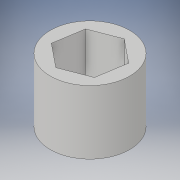
# Autodesk Inventor part: wheel spacer
Saved by Autodesk Inventor 2019 (Build 230136000, 136)
## iProperties
Created: 2019-01-19
Part Number: wheel spacer
Material: Generic
Document SubType Name: Modeling
Designer: Tiberus
Density: 1 g/cm^3
Appearance: Default
Author: Tiberus
Autodesk Inventor part; units mm, degrees
ref_plane "YZ Plane" through (0, 0, 0) normal (1, 0, 0) x (0, 1, 0)
ref_plane "XZ Plane" through (0, 0, 0) normal (0, 1, 0) x (-1, 0, 0)
ref_plane "XY Plane" through (0, 0, 0) normal (0, 0, 1) x (1, 0, 0)
sketch "Sketch1" plane through (0, 0, 0) normal (0, 1, 0) x (-1, 0, 0)
  line L0 (5.8004, -4.6854) -> (-1.1575, -7.366)
  line L1 (-1.1575, -7.366) -> (-6.9579, -2.6806)
  line L2 (-6.9579, -2.6806) -> (-5.8004, 4.6854)
  line L3 (-5.8004, 4.6854) -> (1.1575, 7.366)
  line L4 (1.1575, 7.366) -> (6.9579, 2.6806)
  line L5 (6.9579, 2.6806) -> (5.8004, -4.6854)
  circle A0 centre (0, 0) radius 9.88
  dimension "d0" = 7.366
  constraints: 12 end point, 2 coincident, 1 centre point, 13 other
  measures "d0" vertical distance of L4.end L0.start
extrude "Extrusion1" add sketch "Sketch1" along normal blind 15.875
body "Solid1"
